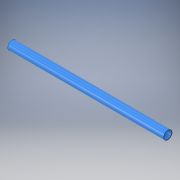
# Autodesk Inventor part: 1in PVC
Saved by Autodesk Inventor 2017 (Build 210142000, 142)
## iProperties
Created: 2017-01-14
Part Number: 1in PVC
Material: PVC-Piping
Document SubType Name: Modeling
Designer: Ben
Density: 1.4 g/cm^3
Appearance: Cyan
Mass: 232.501 g
Surface Area: 1162.72 cm^2
Volume: 166.072 cm^3
Author: Ben
Autodesk Inventor part; units mm, degrees
ref_plane "YZ Plane" through (0, 0, 0) normal (1, 0, 0) x (0, 1, 0)
ref_plane "XZ Plane" through (0, 0, 0) normal (0, 1, 0) x (-1, 0, 0)
ref_plane "XY Plane" through (0, 0, 0) normal (0, 0, 1) x (1, 0, 0)
sketch "Sketch1" plane through (0, 0, 0) normal (1, 0, 0) x (0, 1, 0)
  circle A0 centre (0, 0) radius 16.7005
  circle A1 centre (0, 0) radius 13.8303
  dimension "d0" = 33.401
  dimension "d4" = 2.8702
  constraints: 2 centre point, 2 coincident
  measures "d0" diameter of A0
  measures "d4" radial gap between concentric circles of A0 A1
extrude "Extrusion1" add sketch "Sketch1" along normal mid plane 603.25
body "Solid1"
